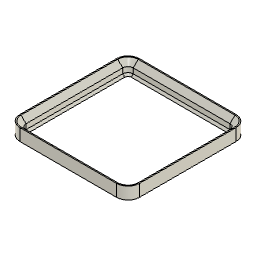
Parametric Gridfinity Baseplate (Autodesk Fusion 360 design; units mm, degrees)
part number: 2025-06-20-10-05-21-198
Autodesk Fusion 360 part; units mm, degrees
sketch "Sketch5" plane through (0, 0, 0) normal (0, 0, 1) x (1, 0, 0)
  line L0 (4, 0) -> (38, 0)
  line L1 (42, 4) -> (42, 38)
  line L2 (38, 42) -> (4, 42)
  line L3 (0, 38) -> (0, 4)
  arc A0 (4, 42) -> (0, 38) centre (4, 38) ccw
  arc A1 (42, 38) -> (38, 42) centre (38, 38) ccw
  arc A2 (38, 0) -> (42, 4) centre (38, 4) ccw
  arc A3 (0, 4) -> (4, 0) centre (4, 4) ccw
  point P0 (42, 0)
  point P1 (0, 42)
  dimension "d20" = 4
  dimension "d21" = 42
  dimension "d22" = 42
  constraint horizontal L0
  constraint vertical L1
  constraint horizontal L2
  constraint vertical L3
  constraint coincident P1 L2
  constraint coincident P1 L3
  constraint tangent L2 A0
  constraint tangent L3 A0
  constraint tangent L1 A1
  constraint tangent L2 A1
  constraint equal A0 A1
  constraint coincident P0 L0
  constraint coincident P0 L1
  constraint tangent L0 A2
  constraint tangent L1 A2
  constraint equal A0 A2
  constraint coincident origin L0
  constraint coincident origin L3
  constraint tangent L0 A3
  constraint tangent L3 A3
  constraint equal A0 A3
  measures "d20" radius of A0
  measures "d21" distance of L0 L2
  measures "d22" distance of L1 L3
extrude "Extrude5" add sketch "Sketch5" along normal blind 4.65 makes body 1
ref_plane "WorkPlane2" through (21, 21, 4.65) normal (0, 0, 1) x (1, 0, 0)
sketch "Sketch6" plane through (0, 0, 4.65) normal (0, 0, 1) x (1, 0, 0)
  arc A0 (0, 4) -> (4, 0) centre (4, 4) ccw
  line L0 (4, 0) -> (38, 0)
  arc A1 (38, 0) -> (42, 4) centre (38, 4) ccw
  line L1 (42, 4) -> (42, 38)
  arc A2 (42, 38) -> (38, 42) centre (38, 38) ccw
  line L2 (38, 42) -> (4, 42)
  arc A3 (4, 42) -> (0, 38) centre (4, 38) ccw
  line L3 (0, 38) -> (0, 4)
extrude "Extrude6" add sketch "Sketch6" against normal blind 2.15 draft -45 separate body makes body 2
extrude "Extrude7" add 1 faces at (14.7167, 26.6667, 2.5) along direction (0, 0, -1) blind 1.8 on bodies 2 bodies 2
extrude "Extrude8" add 1 faces at (14.7167, 26.6667, 0.7) along direction (0, 0, -1) blind 0.7 draft -45 on bodies 2 bodies 2
combine "Combine2" operation cut target body 1 tool bodies 2
pattern_linear "R-Pattern1" count 1 spacing 42 along (0, 1, 0) of 24 faces at (41.0329, 38.2653, 3.6944) (39.85, 15.3333, 1.9) (2.3833, 26.6667, 0.4667) (26.6667, 1.4333, 3.2167) (38.2445, 1.2051, 3.4556) (15.3333, 40.5667, 3.2167) (41.2833, 15.3333, 3.9333) (38.1307, 2.5057, 0.35) (39.6167, 15.3333, 0.4667) (39.4943, 38.1307, 0.35) (15.3333, 39.85, 1.3) (15.3333, 2.6167, 0.2333) (15.3333, 2.15, 1.9) (26.6667, 39.6167, 0.4667) (3.8693, 39.4943, 0.35) (2.1834, 38.3501, 1.3) (38.4362, 2.2021, 1.3) (2.15, 26.6667, 1.9) (2.5057, 3.8693, 0.35) (3.7347, 0.9671, 3.6944) (0.7167, 15.3333, 3.9333) (3.6499, 2.1834, 1.3) (3.7347, 41.0329, 3.6944) (39.4542, 39.1436, 1.3) on bodies 1
ref_plane "WorkPlane3" through (21, 21, 4.25) normal (0, 0, 1) x (1, 0, 0)
split "Split1" by plane through (21, 21, 4.25) normal (0, 0, 1) bodies 1 makes body 3 at (41.7333, 26.6667, 4.3833)
delete_body "RemoveBody1" bodies 3
equation "Rows = 1"
equation "Columns = 1"
equation "U = 42 mm" comment "The base Gridfinity unit size, defaults to 42mm."
equation "d21 = Rows * U"
equation "d22 = Columns * U"
equation "d23 = 2.15 mm + 1.8 mm + 0.7 mm"
equation "d32 = Rows"
equation "d33 = Columns"
equation "d34 = -U"
equation "d35 = U"
named bodies: "Baseplate", "Cutout", "Baseplate (1)"
